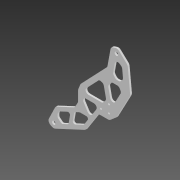
# Autodesk Inventor part: UpperArmBracket
Saved by Autodesk Inventor 2020 (Build 240168000, 168)
## iProperties
Created: 2020-12-02
Part Number: UpperArmBracket
Material: Generic
Document SubType Name: Sheet Metal
Designer: valer
Density: 1 g/cm^3
Sheet Metal Rule: Default
Appearance: Default
Author: valer
Autodesk Inventor part; units mm, degrees
ref_plane "YZ Plane" through (0, 0, 0) normal (1, 0, 0) x (0, 1, 0)
ref_plane "XZ Plane" through (0, 0, 0) normal (0, 1, 0) x (-1, 0, 0)
ref_plane "XY Plane" through (0, 0, 0) normal (0, 0, 1) x (1, 0, 0)
sketch "Base" plane through (0, 0, 0) normal (0, 0, 1) x (1, 0, 0)
  line L0 (9.9216, -55.4575) -> (2.4746, -67.1053)
  line L1 (27.4942, -28.8775) -> (23.6612, -11.0964)
  spline S0 degree 3 poles (23.6612, -11.0964) (23.2667, -9.266) (21.8923, -7.8038) (20.0898, -7.2966) knots 1 1 1 1 2 2 2 2
  line L2 (23.6612, -11.0964) -> (23.2667, -9.266) construction
  line L3 (23.2667, -9.266) -> (21.8923, -7.8038) construction
  line L4 (21.8923, -7.8038) -> (20.0898, -7.2966) construction
  line L5 (20.0898, -7.2966) -> (18.3674, -6.812)
  spline S1 degree 3 poles (18.3674, -6.812) (16.5649, -6.3049) (14.6297, -6.836) (13.3386, -8.1921) knots 3 3 3 3 4 4 4 4
  line L6 (18.3674, -6.812) -> (16.5649, -6.3049) construction
  line L7 (16.5649, -6.3049) -> (14.6297, -6.836) construction
  line L8 (14.6297, -6.836) -> (13.3386, -8.1921) construction
  line L9 (13.3386, -8.1921) -> (-8.2615, -30.8803)
  spline S2 degree 3 poles (-8.2615, -30.8803) (-10.186, -32.9017) (-10.1074, -36.1005) (-8.086, -38.0249) knots 5 5 5 5 6 6 6 6
  line L10 (-8.2615, -30.8803) -> (-10.186, -32.9017) construction
  line L11 (-10.186, -32.9017) -> (-10.1074, -36.1005) construction
  line L12 (-10.1074, -36.1005) -> (-8.086, -38.0249) construction
  spline S3 degree 3 poles (-8.086, -38.0249) (-7.1484, -38.9175) (-5.9041, -39.4163) (-4.6096, -39.4184) knots 6 6 6 6 7 7 7 7
  line L13 (-8.086, -38.0249) -> (-7.1484, -38.9175) construction
  line L14 (-7.1484, -38.9175) -> (-5.9041, -39.4163) construction
  line L15 (-5.9041, -39.4163) -> (-4.6096, -39.4184) construction
  line L16 (-4.6096, -39.4184) -> (18.9386, -39.4565)
  spline S4 degree 3 poles (18.9386, -39.4565) (20.4672, -39.459) (21.9148, -38.7694) (22.8761, -37.5808) knots 8 8 8 8 9 9 9 9
  line L17 (18.9386, -39.4565) -> (20.4672, -39.459) construction
  line L18 (20.4672, -39.459) -> (21.9148, -38.7694) construction
  line L19 (21.9148, -38.7694) -> (22.8761, -37.5808) construction
  line L20 (22.8761, -37.5808) -> (26.4835, -33.1202)
  spline S5 degree 3 poles (26.4835, -33.1202) (27.4448, -31.9316) (27.8164, -30.3718) (27.4942, -28.8775) knots 10 10 10 10 11 11 11 11
  line L21 (26.4835, -33.1202) -> (27.4448, -31.9316) construction
  line L22 (27.4448, -31.9316) -> (27.8164, -30.3718) construction
  line L23 (27.8164, -30.3718) -> (27.4942, -28.8775) construction
  line L24 (48.076, 1.4731) -> (40.4011, 1.4855)
  spline S6 degree 3 poles (40.4011, 1.4855) (38.8725, 1.488) (37.4249, 0.7984) (36.4636, -0.3902) knots 1 1 1 1 2 2 2 2
  line L25 (40.4011, 1.4855) -> (38.8725, 1.488) construction
  line L26 (38.8725, 1.488) -> (37.4249, 0.7984) construction
  line L27 (37.4249, 0.7984) -> (36.4636, -0.3902) construction
  line L28 (36.4636, -0.3902) -> (32.8562, -4.8508)
  spline S7 degree 3 poles (32.8562, -4.8508) (31.8949, -6.0394) (31.5233, -7.5992) (31.8455, -9.0935) knots 3 3 3 3 4 4 4 4
  line L29 (32.8562, -4.8508) -> (31.8949, -6.0394) construction
  line L30 (31.8949, -6.0394) -> (31.5233, -7.5992) construction
  line L31 (31.5233, -7.5992) -> (31.8455, -9.0935) construction
  line L32 (31.8455, -9.0935) -> (35.2347, -24.8159)
  spline S8 degree 3 poles (35.2347, -24.8159) (35.8228, -27.5442) (38.5113, -29.2792) (41.2397, -28.691) knots 5 5 5 5 6 6 6 6
  line L33 (35.2347, -24.8159) -> (35.8228, -27.5442) construction
  line L34 (35.8228, -27.5442) -> (38.5113, -29.2792) construction
  line L35 (38.5113, -29.2792) -> (41.2397, -28.691) construction
  spline S9 degree 3 poles (41.2397, -28.691) (42.6921, -28.3779) (43.9332, -27.4415) (44.6329, -26.1307) knots 6 6 6 6 7 7 7 7
  line L36 (41.2397, -28.691) -> (42.6921, -28.3779) construction
  line L37 (42.6921, -28.3779) -> (43.9332, -27.4415) construction
  line L38 (43.9332, -27.4415) -> (44.6329, -26.1307) construction
  line L39 (44.6329, -26.1307) -> (54.0451, -8.4978)
  spline S10 degree 3 poles (54.0451, -8.4978) (54.8805, -6.9328) (54.8341, -5.0444) (53.9229, -3.5223) knots 8 8 8 8 9 9 9 9
  line L40 (54.0451, -8.4978) -> (54.8805, -6.9328) construction
  line L41 (54.8805, -6.9328) -> (54.8341, -5.0444) construction
  line L42 (54.8341, -5.0444) -> (53.9229, -3.5223) construction
  line L43 (53.9229, -3.5223) -> (52.4037, -0.9847)
  spline S11 degree 3 poles (52.4037, -0.9847) (51.4925, 0.5374) (49.8499, 1.4702) (48.076, 1.4731) knots 10 10 10 10 11 11 11 11
  line L44 (52.4037, -0.9847) -> (51.4925, 0.5374) construction
  line L45 (51.4925, 0.5374) -> (49.8499, 1.4702) construction
  line L46 (49.8499, 1.4702) -> (48.076, 1.4731) construction
  line L47 (-21.9472, -75.7228) -> (-28.6399, -78.8304)
  spline S12 degree 3 poles (-28.6399, -78.8304) (-29.5745, -79.2644) (-30.2387, -80.1271) (-30.4193, -81.1416) knots 1 1 1 1 2 2 2 2
  line L48 (-28.6399, -78.8304) -> (-29.5745, -79.2644) construction
  line L49 (-29.5745, -79.2644) -> (-30.2387, -80.1271) construction
  line L50 (-30.2387, -80.1271) -> (-30.4193, -81.1416) construction
  line L51 (-30.4193, -81.1416) -> (-32.8551, -94.8265)
  spline S13 degree 3 poles (-32.8551, -94.8265) (-33.1608, -96.5439) (-32.0164, -98.1839) (-30.299, -98.4896) knots 3 3 3 3 4 4 4 4
  line L52 (-32.8551, -94.8265) -> (-33.1608, -96.5439) construction
  line L53 (-33.1608, -96.5439) -> (-32.0164, -98.1839) construction
  line L54 (-32.0164, -98.1839) -> (-30.299, -98.4896) construction
  spline S14 degree 3 poles (-30.299, -98.4896) (-29.6609, -98.6032) (-29.0032, -98.5177) (-28.4153, -98.2447) knots 4 4 4 4 5 5 5 5
  line L55 (-30.299, -98.4896) -> (-29.6609, -98.6032) construction
  line L56 (-29.6609, -98.6032) -> (-29.0032, -98.5177) construction
  line L57 (-29.0032, -98.5177) -> (-28.4153, -98.2447) construction
  line L58 (-28.4153, -98.2447) -> (-13.6329, -91.3807)
  spline S15 degree 3 poles (-13.6329, -91.3807) (-13.0876, -91.1275) (-12.6259, -90.7239) (-12.3021, -90.2173) knots 6 6 6 6 7 7 7 7
  line L59 (-13.6329, -91.3807) -> (-13.0876, -91.1275) construction
  line L60 (-13.0876, -91.1275) -> (-12.6259, -90.7239) construction
  line L61 (-12.6259, -90.7239) -> (-12.3021, -90.2173) construction
  line L62 (-12.3021, -90.2173) -> (-5.6517, -79.8155)
  spline S16 degree 3 poles (-5.6517, -79.8155) (-4.712, -78.3458) (-5.1417, -76.3927) (-6.6114, -75.4531) knots 8 8 8 8 9 9 9 9
  line L63 (-5.6517, -79.8155) -> (-4.712, -78.3458) construction
  line L64 (-4.712, -78.3458) -> (-5.1417, -76.3927) construction
  line L65 (-5.1417, -76.3927) -> (-6.6114, -75.4531) construction
  spline S17 degree 3 poles (-6.6114, -75.4531) (-7.1179, -75.1292) (-7.7064, -74.9567) (-8.3076, -74.9557) knots 9 9 9 9 10 10 10 10
  line L66 (-6.6114, -75.4531) -> (-7.1179, -75.1292) construction
  line L67 (-7.1179, -75.1292) -> (-7.7064, -74.9567) construction
  line L68 (-7.7064, -74.9567) -> (-8.3076, -74.9557) construction
  line L69 (-8.3076, -74.9557) -> (-18.3864, -74.9394)
  spline S18 degree 3 poles (-18.3864, -74.9394) (-19.6163, -74.9374) (-20.8317, -75.2048) (-21.9472, -75.7228) knots 11 11 11 11 12 12 12 12
  line L70 (-18.3864, -74.9394) -> (-19.6163, -74.9374) construction
  line L71 (-19.6163, -74.9374) -> (-20.8317, -75.2048) construction
  line L72 (-20.8317, -75.2048) -> (-21.9472, -75.7228) construction
  line L73 (-48.3702, -107.5105) -> (-42.1242, -104.6103)
  spline S19 degree 3 poles (-42.1242, -104.6103) (-41.1895, -104.1763) (-40.5254, -103.3136) (-40.3448, -102.2991) knots 1 1 1 1 2 2 2 2
  line L74 (-42.1242, -104.6103) -> (-41.1895, -104.1763) construction
  line L75 (-41.1895, -104.1763) -> (-40.5254, -103.3136) construction
  line L76 (-40.5254, -103.3136) -> (-40.3448, -102.2991) construction
  line L77 (-40.3448, -102.2991) -> (-37.9089, -88.6141)
  spline S20 degree 3 poles (-37.9089, -88.6141) (-37.6032, -86.8968) (-38.7476, -85.2567) (-40.465, -84.9511) knots 3 3 3 3 4 4 4 4
  line L78 (-37.9089, -88.6141) -> (-37.6032, -86.8968) construction
  line L79 (-37.6032, -86.8968) -> (-38.7476, -85.2567) construction
  line L80 (-38.7476, -85.2567) -> (-40.465, -84.9511) construction
  spline S21 degree 3 poles (-40.465, -84.9511) (-41.1032, -84.8375) (-41.7608, -84.923) (-42.3487, -85.196) knots 4 4 4 4 5 5 5 5
  line L81 (-40.465, -84.9511) -> (-41.1032, -84.8375) construction
  line L82 (-41.1032, -84.8375) -> (-41.7608, -84.923) construction
  line L83 (-41.7608, -84.923) -> (-42.3487, -85.196) construction
  line L84 (-42.3487, -85.196) -> (-55.62, -91.3583)
  spline S22 degree 3 poles (-55.62, -91.3583) (-58.5888, -92.7369) (-60.4901, -95.7106) (-60.4954, -98.9839) knots 6 6 6 6 7 7 7 7
  line L85 (-55.62, -91.3583) -> (-58.5888, -92.7369) construction
  line L86 (-58.5888, -92.7369) -> (-60.4901, -95.7106) construction
  line L87 (-60.4901, -95.7106) -> (-60.4954, -98.9839) construction
  line L88 (-60.4954, -98.9839) -> (-60.5001, -101.8743)
  spline S23 degree 3 poles (-60.5001, -101.8743) (-60.5016, -102.8275) (-60.0726, -103.7303) (-59.3327, -104.3312) knots 8 8 8 8 9 9 9 9
  line L89 (-60.5001, -101.8743) -> (-60.5016, -102.8275) construction
  line L90 (-60.5016, -102.8275) -> (-60.0726, -103.7303) construction
  line L91 (-60.0726, -103.7303) -> (-59.3327, -104.3312) construction
  line L92 (-59.3327, -104.3312) -> (-54.3872, -108.3475)
  spline S24 degree 3 poles (-54.3872, -108.3475) (-53.4505, -109.1083) (-52.1622, -109.2688) (-51.0675, -108.7612) knots 10 10 10 10 11 11 11 11
  line L93 (-54.3872, -108.3475) -> (-53.4505, -109.1083) construction
  line L94 (-53.4505, -109.1083) -> (-52.1622, -109.2688) construction
  line L95 (-52.1622, -109.2688) -> (-51.0675, -108.7612) construction
  line L96 (-51.0675, -108.7612) -> (-48.3702, -107.5105)
  spline S25 degree 3 poles (47.0119, 38.1138) (45.2288, 37.5547) (43.8998, 36.0574) (43.5563, 34.2206) knots 0 0 0 0 1 1 1 1
  line L97 (47.0119, 38.1138) -> (45.2288, 37.5547) construction
  line L98 (45.2288, 37.5547) -> (43.8998, 36.0574) construction
  line L99 (43.8998, 36.0574) -> (43.5563, 34.2206) construction
  line L100 (43.5563, 34.2206) -> (40.6068, 18.4492)
  spline S26 degree 3 poles (40.6068, 18.4492) (40.3308, 16.9732) (40.7254, 15.451) (41.6836, 14.295) knots 2 2 2 2 3 3 3 3
  line L101 (40.6068, 18.4492) -> (40.3308, 16.9732) construction
  line L102 (40.3308, 16.9732) -> (40.7254, 15.451) construction
  line L103 (40.7254, 15.451) -> (41.6836, 14.295) construction
  line L104 (41.6836, 14.295) -> (43.8143, 11.7247)
  spline S27 degree 3 poles (43.8143, 11.7247) (44.7726, 10.5687) (46.1953, 9.8987) (47.6968, 9.8963) knots 4 4 4 4 5 5 5 5
  line L105 (43.8143, 11.7247) -> (44.7726, 10.5687) construction
  line L106 (44.7726, 10.5687) -> (46.1953, 9.8987) construction
  line L107 (46.1953, 9.8987) -> (47.6968, 9.8963) construction
  line L108 (47.6968, 9.8963) -> (50.8215, 9.8912)
  spline S28 degree 3 poles (50.8215, 9.8912) (52.2537, 9.8889) (53.6196, 10.4944) (54.5797, 11.5572) knots 6 6 6 6 7 7 7 7
  line L109 (50.8215, 9.8912) -> (52.2537, 9.8889) construction
  line L110 (52.2537, 9.8889) -> (53.6196, 10.4944) construction
  line L111 (53.6196, 10.4944) -> (54.5797, 11.5572) construction
  line L112 (54.5797, 11.5572) -> (57.23, 14.4911)
  spline S29 degree 3 poles (57.23, 14.4911) (58.19, 15.5539) (58.6541, 16.9742) (58.5067, 18.3988) knots 8 8 8 8 9 9 9 9
  line L113 (57.23, 14.4911) -> (58.19, 15.5539) construction
  line L114 (58.19, 15.5539) -> (58.6541, 16.9742) construction
  line L115 (58.6541, 16.9742) -> (58.5067, 18.3988) construction
  line L116 (58.5067, 18.3988) -> (58.5067, 18.3988) construction
  line L117 (58.5067, 18.3988) -> (57.0665, 32.3174) construction
  line L118 (57.0665, 32.3174) -> (57.0665, 32.3174) construction
  spline S30 degree 3 poles (57.0665, 32.3174) (56.9104, 33.8263) (56.0847, 35.1852) (54.8175, 36.019) knots 10 10 10 10 11 11 11 11
  line L119 (57.0665, 32.3174) -> (56.9104, 33.8263) construction
  line L120 (56.9104, 33.8263) -> (56.0847, 35.1852) construction
  line L121 (56.0847, 35.1852) -> (54.8175, 36.019) construction
  line L122 (54.8175, 36.019) -> (52.1444, 37.7777)
  spline S31 degree 3 poles (52.1444, 37.7777) (50.8772, 38.6115) (49.3024, 38.8319) (47.8549, 38.3781) knots 12 12 12 12 13 13 13 13
  line L123 (52.1444, 37.7777) -> (50.8772, 38.6115) construction
  line L124 (50.8772, 38.6115) -> (49.3024, 38.8319) construction
  line L125 (49.3024, 38.8319) -> (47.8549, 38.3781) construction
  line L126 (47.8549, 38.3781) -> (47.0119, 38.1138)
  line L127 (-23.1618, -60.4945) -> (-29.5284, -71.8657)
  line L128 (-29.5284, -71.8657) -> (-62.1902, -87.0318)
  spline S32 degree 3 poles (-62.1902, -87.0318) (-63.5183, -87.6485) (-64.5909, -88.7074) (-65.2246, -90.0275) knots 2 2 2 2 3 3 3 3
  line L129 (-62.1902, -87.0318) -> (-63.5183, -87.6485) construction
  line L130 (-63.5183, -87.6485) -> (-64.5909, -88.7074) construction
  line L131 (-64.5909, -88.7074) -> (-65.2246, -90.0275) construction
  line L132 (-65.2246, -90.0275) -> (-76.3276, -113.1575)
  spline S33 degree 3 poles (-76.3276, -113.1575) (-77.8374, -116.3026) (-76.5116, -120.0762) (-73.3665, -121.5859) knots 4 4 4 4 5 5 5 5
  line L133 (-76.3276, -113.1575) -> (-77.8374, -116.3026) construction
  line L134 (-77.8374, -116.3026) -> (-76.5116, -120.0762) construction
  line L135 (-76.5116, -120.0762) -> (-73.3665, -121.5859) construction
  line L136 (-73.3665, -121.5859) -> (-70.2747, -123.0701)
  spline S34 degree 3 poles (-70.2747, -123.0701) (-68.5722, -123.8873) (-66.5934, -123.9) (-64.8806, -123.1047) knots 6 6 6 6 7 7 7 7
  line L137 (-70.2747, -123.0701) -> (-68.5722, -123.8873) construction
  line L138 (-68.5722, -123.8873) -> (-66.5934, -123.9) construction
  line L139 (-66.5934, -123.9) -> (-64.8806, -123.1047) construction
  line L140 (-64.8806, -123.1047) -> (-11.4397, -98.2899)
  spline S35 degree 3 poles (-11.4397, -98.2899) (-10.3491, -97.7835) (-9.4257, -96.9763) (-8.778, -95.9633) knots 8 8 8 8 9 9 9 9
  line L141 (-11.4397, -98.2899) -> (-10.3491, -97.7835) construction
  line L142 (-10.3491, -97.7835) -> (-9.4257, -96.9763) construction
  line L143 (-9.4257, -96.9763) -> (-8.778, -95.9633) construction
  line L144 (-8.778, -95.9633) -> (13.8923, -60.5048)
  line L145 (13.8923, -60.5048) -> (33.6904, -60.5368)
  line L146 (33.6904, -60.5368) -> (45.5763, -50.449)
  spline S36 degree 3 poles (45.5763, -50.449) (46.0948, -49.9698) (46.5294, -49.4071) (46.8618, -48.7842) knots 15 15 15 15 16 16 16 16
  line L147 (45.5763, -50.449) -> (46.0948, -49.9698) construction
  line L148 (46.0948, -49.9698) -> (46.5294, -49.4071) construction
  line L149 (46.5294, -49.4071) -> (46.8618, -48.7842) construction
  line L150 (46.8618, -48.7842) -> (70.7777, -3.9802)
  spline S37 degree 3 poles (70.7777, -3.9802) (71.3704, -2.8697) (71.6179, -1.6075) (71.4912, -0.3555) knots 17 17 17 17 18 18 18 18
  line L151 (70.7777, -3.9802) -> (71.3704, -2.8697) construction
  line L152 (71.3704, -2.8697) -> (71.6179, -1.6075) construction
  line L153 (71.6179, -1.6075) -> (71.4912, -0.3555) construction
  line L154 (71.4912, -0.3555) -> (67.2665, 40.4746)
  spline S38 degree 3 poles (67.2665, 40.4746) (67.1098, 41.9895) (66.411, 43.3968) (65.2988, 44.4374) knots 19 19 19 19 20 20 20 20
  line L155 (67.2665, 40.4746) -> (67.1098, 41.9895) construction
  line L156 (67.1098, 41.9895) -> (66.411, 43.3968) construction
  line L157 (66.411, 43.3968) -> (65.2988, 44.4374) construction
  line L158 (65.2988, 44.4374) -> (51.2619, 57.5695)
  spline S39 degree 3 poles (51.2619, 57.5695) (49.5995, 59.1247) (47.2288, 59.6652) (45.0565, 58.9842) knots 21 21 21 21 22 22 22 22
  line L159 (51.2619, 57.5695) -> (49.5995, 59.1247) construction
  line L160 (49.5995, 59.1247) -> (47.2288, 59.6652) construction
  line L161 (47.2288, 59.6652) -> (45.0565, 58.9842) construction
  line L162 (45.0565, 58.9842) -> (40.1382, 57.4422)
  spline S40 degree 3 poles (40.1382, 57.4422) (37.9094, 56.7434) (36.2481, 54.8717) (35.8188, 52.5758) knots 23 23 23 23 24 24 24 24
  line L163 (40.1382, 57.4422) -> (37.9094, 56.7434) construction
  line L164 (37.9094, 56.7434) -> (36.2481, 54.8717) construction
  line L165 (36.2481, 54.8717) -> (35.8188, 52.5758) construction
  line L166 (35.8188, 52.5758) -> (30.3576, 23.374)
  spline S41 degree 3 poles (30.3576, 23.374) (30.1331, 22.1736) (29.5655, 21.064) (28.7235, 20.1795) knots 25 25 25 25 26 26 26 26
  line L167 (30.3576, 23.374) -> (30.1331, 22.1736) construction
  line L168 (30.1331, 22.1736) -> (29.5655, 21.064) construction
  line L169 (29.5655, 21.064) -> (28.7235, 20.1795) construction
  line L170 (28.7235, 20.1795) -> (-23.1301, -34.286)
  line L171 (-9.0955, -47.8337) -> (5.7681, -47.8577)
  line L172 (-13.2723, -55.4219) -> (-5.8556, -67.0937)
  line L173 (57.0665, 32.3174) -> (58.5067, 18.3988)
  arc A0 (-9.0955, -47.8337) -> (-13.2723, -55.4219) centre (-9.1035, -52.7729) ccw
  arc A1 (9.9216, -55.4575) -> (5.7681, -47.8577) centre (5.7602, -52.7969) ccw
  arc A2 (-5.8556, -67.0937) -> (2.4746, -67.1053) centre (-1.6868, -64.4447) ccw
  circle A3 centre (-67.5276, -114.948) radius 3.175
  circle A4 centre (46.408, 50.5954) radius 3.175
  line L174 (-23.1618, -60.4945) -> (-23.1301, -34.286)
  point P0 (0, 0)
  dimension "d10" = 6.35
  dimension "d11" = 6.35
  measures "d10" diameter of A3
  measures "d11" diameter of A4
extrude "Plate1" add sketch "Base" along normal blind 3.175
chamfer "ChamferFeature" distance 6.35 angle 45 1 edges at (-23.1301, -34.286, 1.5875)
fillet "FilletFeature" radius 6.35 6 edges at (-18.7516, -29.687, 1.5875) (-23.1378, -40.636, 1.5875) (-23.1618, -60.4945, 1.5875) (-29.5284, -71.8657, 1.5875) (33.6904, -60.5368, 1.5875) (13.8923, -60.5048, 1.5875)
sketch "MountHoles" plane through (0, 0, 0) normal (0, 0, -1) x (-1, 0, 0)
  circle A0 centre (-18.3798, -50.1232) radius 2.2451
  circle A1 centre (-32.8758, -50.1232) radius 2.2451
  line L0 (-18.3798, -50.1232) -> (-9.9131, -50.1232) construction
  arc A2 (-5.7681, -47.8577) -> (-9.9216, -55.4575) centre (-5.7602, -52.7969) ccw construction
  line L1 (-18.3798, -50.1232) -> (-32.8758, -50.1232) construction
  line L2 (-35.4724, -59.0244) -> (-45.5763, -50.449) projected
  line L3 (-5.7681, -47.8577) -> (-47.3205, -47.9249) construction
  line L4 (-70.7777, -3.9802) -> (-46.8618, -48.7842) projected
  line L5 (-5.7681, -47.8577) -> (9.0955, -47.8337) construction
  circle A3 centre (-32.8993, -35.6272) radius 2.2451
  line L6 (-32.8993, -35.6272) -> (-18.3798, -50.1232) construction
  line L7 (-32.8758, -50.1232) -> (-32.8993, -35.6272) construction
  point P0 (0, 0)
  dimension "d16" = 4.4901
  dimension "d18" = 8.4667
  dimension "d19" = 8.4667
  constraints: 10 end point, 3 centre point, 2 collinear, 2 equal radius, 1 equal length, 1 horizontal, 1 perpendicular, 1 point on circle, 1 point on line, 1 tangent
  measures "d16" diameter of A0
  measures "d18" distance of L0.start L0.end
  measures "d19" distance from line of L2 L1.end
hole "MountHolesFeature" at (32.8758, -50.1232, 0) at (18.3798, -50.1232, 0) at (32.8993, -35.6272, 0) direction (0, 0, 1) diameter 3.175 end through all
equation "\"d25\" = Thickness"
equation "\"d4\" = Thickness"
equation "\"BendRadius\" = Thickness"
equation "\"BendReliefWidth\" = Thickness"
equation "\"BendReliefDepth\" = 0.5 * Thickness"
equation "\"CornerReliefSize\" = 4 * Thickness"
equation "\"MinimumRemnant\" = 2 * Thickness"
equation "\"TransitionRadius\" = BendRadius"
equation "\"JacobiRadiusSize\" = BendRadius"
equation "\"GapSize\" = Thickness"
equation "\"Thickness\" = 3.175"
body "Solid1"
